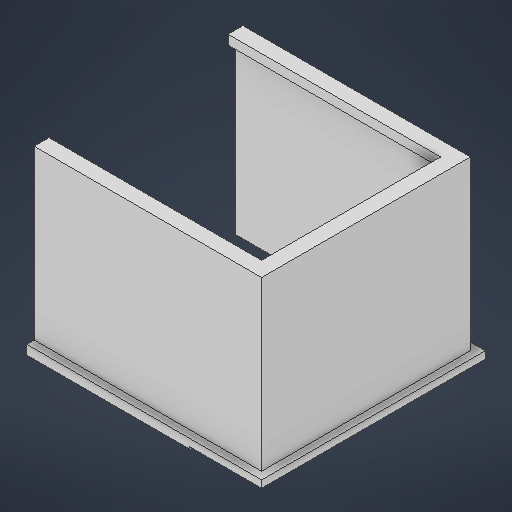
# Autodesk Inventor part: Galvo Housing-01
Saved by Autodesk Inventor 2025 (Build 290162000, 162)
## iProperties
Created: 2024-06-12
Part Number: Galvo Housing-01
Material: Generic
Document SubType Name: Modeling
Designer: mayhe
Density: 1 g/cm^3
Appearance: Default
Author: mayhe
Autodesk Inventor part; units mm, degrees
ref_plane "YZ Plane" through (0, 0, 0) normal (1, 0, 0) x (0, 1, 0)
ref_plane "XZ Plane" through (0, 0, 0) normal (0, 1, 0) x (-1, 0, 0)
ref_plane "XY Plane" through (0, 0, 0) normal (0, 0, 1) x (1, 0, 0)
sketch "Sketch8" plane through (0, 0, 0) normal (0, 1, 0) x (-1, 0, 0)
  line L0 (-61, -56) -> (61, -56)
  line L1 (61, -56) -> (61, 56)
  line L2 (61, 56) -> (-61, 56)
  line L3 (-61, 56) -> (-61, -56)
  line L4 (-61, -56) -> (61, 56) construction
  line L5 (61, -56) -> (-61, 56) construction
  point P0 (0, 0)
  dimension "d26" = 122
  dimension "d27" = 112
  constraints: 12 end point, 2 midpoint, 2 parallel, 1 horizontal, 1 perpendicular
  measures "d26" distance of L2.end L1.end
  measures "d27" distance of L1.end L0.end
extrude "Extrusion7" add sketch "Sketch8" along normal blind 95
sketch "Sketch9" plane through (0, 0, 0) normal (0, -1, 0) x (1, 0, 0)
  line L0 (-61, 56) -> (61, 56) projected
  line L1 (-61, -56) -> (61, -56)
  line L2 (61, -56) -> (61, 56)
  line L3 (61, 56) -> (-61, 56)
  line L4 (-61, 56) -> (-61, -56)
  line L5 (-61, -56) -> (61, 56) construction
  line L6 (61, -56) -> (-61, 56) construction
  line L7 (57, 52) -> (57, -52)
  line L8 (57, -52) -> (-61, -52)
  line L9 (-61, 52) -> (57, 52)
  line L10 (53, -48) -> (53, 48)
  line L11 (53, 48) -> (-61, 48)
  line L12 (-61, -48) -> (53, -48)
  line L13 (-58.8844, -52) -> (-58.8844, -54.0578)
  line L14 (-58.8844, 54.0578) -> (-58.8844, 52)
  line L15 (-54.6854, 48) -> (-54.6854, 50.203)
  line L16 (-54.6854, -50.203) -> (-54.6854, -48)
  point P0 (0, 0)
  dimension "d30" = 4
  dimension "d31" = 4
  dimension "d47" = 4
  dimension "d48" = 4
  dimension "d49" = 4
  dimension "d50" = 4
  constraints: 32 end point, 12 point on line, 8 parallel, 3 perpendicular, 2 midpoint, 1 horizontal
  measures "d30" distance between parallel lines of L2 L7
  measures "d31" distance between parallel lines of L7 L10
  measures "d47" distance between parallel lines of L0 L9
  measures "d48" distance between parallel lines of L11 L9
  measures "d49" distance between parallel lines of L1 L8
  measures "d50" distance between parallel lines of L8 L12
extrude "Extrusion8" cut sketch "Sketch9" against normal blind 115 contours L11 L10 L12 L4
extrude "Extrusion9" cut sketch "Sketch9" against normal blind 90 contours L9 L7 L8 L4 L12 L10 L11
sketch "Sketch10" plane through (0, 0, 0) normal (0, -1, 0) x (1, 0, 0)
  line L0 (61, -56) -> (-61, -56)
  line L1 (-61, -56) -> (-61, 56)
  line L2 (-61, 56) -> (61, 56)
  line L3 (61, 56) -> (61, -56)
  line L4 (61, -56) -> (-61, 56) construction
  line L5 (-61, -56) -> (61, 56) construction
  line L6 (-65, 60) -> (-65, -60)
  line L7 (-65, -60) -> (65, -60)
  line L8 (65, -60) -> (65, 60)
  line L9 (65, 60) -> (-65, 60)
  line L10 (-61, 56) -> (-65, 56)
  line L11 (-61, -56) -> (-65, -56)
  line L12 (-61, 56) -> (-61, 60)
  line L13 (-61, -56) -> (-61, -60)
  point P0 (0, 0)
  dimension "d36" = 4
  constraints: 28 end point, 5 perpendicular, 5 point on line, 4 parallel, 2 midpoint, 1 horizontal, 3 other
  measures "d36" distance between parallel lines of L1 L6
extrude "Extrusion10" add sketch "Sketch10" against normal blind 5 contours L3 L2 L12 L9 L8 L7 L13 L0
sketch "Sketch11" plane through (0, 0, 0) normal (0, -1, 0) x (1, 0, 0)
  circle A0 centre (-71, 9) radius 135
  line L0 (57, 52) -> (57, -52) projected
  line L1 (65, -60) -> (65, 60) projected
  circle A1 centre (-71, 9) radius 110
  line L2 (14.668, -60) -> (65, -60)
  line L3 (65, -60) -> (65, 60)
  line L4 (65, 60) -> (26.4628, 60)
  line L5 (-61, 60) -> (65, 60) projected
  point P0 (0, 0)
  dimension "d39" = 270
  dimension "d41" = 136
  dimension "d42" = 220
  constraints: 6 end point, 2 centre point, 2 point on circle, 1 coincident, 1 collinear, 1 perpendicular, 1 point on line
  measures "d39" diameter of A0
  measures "d41" distance from line of L1 A0.centre
  measures "d42" diameter of A1
extrude "Extrusion11" cut sketch "Sketch11" against normal blind 1.125 contours A0 L0 | A0 L4 L1 L2 | L0 A0 L2 A1 L4
body "Solid3"
